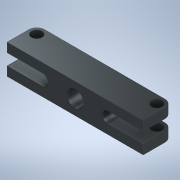
# Autodesk Inventor part: Practica 7
Saved by Autodesk Inventor 2020.2 (Build 242310000, 310)
## iProperties
Created: 2020-02-16
Part Number: Practica 7
Material: Hierro, gris
Document SubType Name: Chapa
Designer: Luis Gallardo
Density: 7.15 g/cm^3
Sheet Metal Rule: Por defecto_mm
Appearance: Gris hierro
Author: Luis Gallardo
Autodesk Inventor part; units mm, degrees
ref_plane "YZ Plane" through (0, 0, 0) normal (1, 0, 0) x (0, 1, 0)
ref_plane "XZ Plane" through (0, 0, 0) normal (0, 1, 0) x (-1, 0, 0)
ref_plane "XY Plane" through (0, 0, 0) normal (0, 0, 1) x (1, 0, 0)
sketch "Boceto1" plane through (0, 0, 0) normal (0, 1, 0) x (-1, 0, 0)
  line L0 (0, 0) -> (-102, 0)
  line L1 (-102, 0) -> (-102, -16.2)
  line L2 (-96, -22.2) -> (-6, -22.2)
  line L3 (0, -16.2) -> (0, 0)
  arc A0 (-102, -16.2) -> (-96, -22.2) centre (-96, -16.2) ccw
  arc A1 (-6, -22.2) -> (0, -16.2) centre (-6, -16.2) ccw
  line L4 (0, 0) -> (-51, 0) construction
  line L5 (-51, 0) -> (-51, -11.1) construction
  circle A2 centre (-6, -16.2) radius 4
  circle A3 centre (-96, -16.2) radius 4
  dimension "d0" = 6
  dimension "d1" = 102
  dimension "d2" = 22.2
  dimension "d3" = 51
  dimension "d4" = 11.1
  dimension "d5" = 8
  dimension "d6" = 8
  constraints: 12 end point, 4 centre point, 4 perpendicular, 4 point on circle, 4 tangent, 2 coincident, 1 equal radius, 1 horizontal, 1 midpoint
  measures "d0" radius of A0
  measures "d1" distance of L0.start L0.end
  measures "d2" distance between parallel lines of L2 L0
  measures "d3" distance of L0.start L4.end
  measures "d4" distance of L4.end L5.end
  measures "d5" diameter of A2
  measures "d6" diameter of A3
extrude "Extrusión1" add sketch "Boceto1" along normal blind 22.2 contours L3 A1 L2 A0 L1 L0 | A2 | A3
sketch "Boceto2" plane through (0, 22.2, 0) normal (0, 1, 0) x (1, 0, 0)
  arc A0 (6, 22.2) -> (0, 16.2) centre (6, 16.2) ccw projected
  circle A1 centre (6, 16.2) radius 4
  arc A2 (102, 16.2) -> (96, 22.2) centre (96, 16.2) ccw projected
  circle A3 centre (96, 16.2) radius 4
  point P0 (0, 0)
  dimension "d9" = 8
  dimension "d10" = 8
  constraints: 2 centre point, 2 coincident
  measures "d9" diameter of A1
  measures "d10" diameter of A3
extrude "Extrusión2" cut sketch "Boceto2" against normal through all
sketch "Boceto3" plane through (96, 0, -22.2) normal (0, 0, -1) x (-1, 0, 0)
  line L0 (-6, 0) -> (-6, 22.2) projected
  line L1 (96, 0) -> (96, 22.2) projected
  line L2 (0, 0) -> (90, 0) projected
  line L3 (0, 22.2) -> (90, 22.2) projected
  line L4 (96, 22.2) -> (90, 22.2) projected
  line L5 (96, 0) -> (90, 0) projected
  line L6 (0, 0) -> (-6, 0) projected
  line L7 (0, 22.2) -> (-6, 22.2) projected
  line L8 (-6, 0) -> (45, 0) construction
  line L9 (45, 0) -> (45, 11.1) construction
  arc A0 (69.44, 15.35) -> (69.44, 6.85) centre (69.44, 11.1) ccw
  line L10 (69.44, 6.85) -> (96, 6.85)
  line L11 (96, 15.35) -> (69.44, 15.35)
  arc A1 (20.56, 6.85) -> (20.56, 15.35) centre (20.56, 11.1) ccw
  line L12 (20.56, 6.85) -> (-6, 6.85)
  line L13 (-6, 15.35) -> (20.56, 15.35)
  circle A2 centre (45, 11.1) radius 6.25
  dimension "d13" = 51
  dimension "d14" = 11.1
  dimension "d15" = 8.5
  dimension "d16" = 26.56
  dimension "d17" = 12.5
  constraints: 12 end point, 5 symmetric about line, 4 point on circle, 3 centre point, 2 point on line, 1 coincident, 1 horizontal, 1 midpoint, 1 perpendicular, 1 tangent, 1 other
  measures "d13" distance of L0.start L8.end
  measures "d14" distance of L8.end L9.end
  measures "d15" diameter of A0
  measures "d16" distance from line of L1 A0.centre
  measures "d17" diameter of A2
extrude "Extrusión3" cut sketch "Boceto3" against normal through all contours L0 L13 A1 L12 | L10 A0 L11 L1 | A2
equation "\"Radio_pliegue\" = Grosor"
equation "\"Anchura_desahogo_plegado\" = Grosor"
equation "\"Profundidad_desahogo_plegado\" = 0.5 * Grosor"
equation "\"Tamaño_destalonado\" = 4 * Grosor"
equation "\"Remanente_mínimo\" = 2 * Grosor"
equation "\"Radiodetransición\" = Radio_pliegue"
equation "\"Tamaño_de_radio_de_Jacobi\" = Radio_pliegue"
equation "\"TamañoSeparación\" = Grosor"
equation "\"Grosor\" = 0.5"
